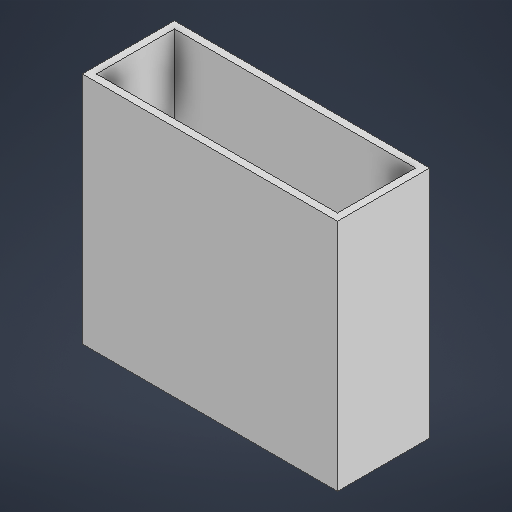
# Autodesk Inventor part: five_cell_bottom_case
Saved by Autodesk Inventor 2026 (Build 300175050, 175E)
## iProperties
Created: 2025-06-13
Part Number: five_cell_bottom_case
Material: Generic
Document SubType Name: Modeling
Designer: hamth
Density: 1 g/cm^3
Appearance: Default
Author: hamth
Autodesk Inventor part; units mm, degrees
ref_plane "YZ Plane" through (0, 0, 0) normal (1, 0, 0) x (0, 1, 0)
ref_plane "XZ Plane" through (0, 0, 0) normal (0, 1, 0) x (-1, 0, 0)
ref_plane "XY Plane" through (0, 0, 0) normal (0, 0, 1) x (1, 0, 0)
sketch "Sketch1" plane through (0, 0, 0) normal (0, 1, 0) x (-1, 0, 0)
  line L0 (57.7037, 0.576) -> (-56.5963, 0.576)
  line L1 (-56.5963, 0.576) -> (-56.5963, 41.851)
  line L2 (-56.5963, 41.851) -> (57.7037, 41.851)
  line L3 (57.7037, 41.851) -> (57.7037, 0.576)
  point P0 (0, 0)
  dimension "d0" = 114.3
  dimension "d1" = 41.275
  constraints: 8 end point, 2 parallel, 1 horizontal, 1 perpendicular
  measures "d0" distance of L1.end L2.end
  measures "d1" distance of L2.end L0.start
extrude "Extrusion1" add sketch "Sketch1" along normal blind 3.175
sketch "Sketch2" plane through (0, 3.175, 0) normal (0, 1, 0) x (1, 0, 0)
  line L0 (56.5963, -0.576) -> (-57.7037, -0.576) projected
  line L1 (-57.7037, -0.576) -> (56.5963, -0.576)
  line L2 (56.5963, -0.576) -> (56.5963, -3.751)
  line L3 (56.5963, -3.751) -> (-57.7037, -3.751)
  line L4 (-57.7037, -3.751) -> (-57.7037, -0.576)
  point P0 (0, 0)
  dimension "d4" = 3.175
  dimension "d5" = 114.3
  constraints: 8 end point, 2 parallel, 1 perpendicular, 1 point on line
  measures "d4" distance of L1.end L2.end
  measures "d5" distance of L2.end L3.end
extrude "Extrusion2" add sketch "Sketch2" along normal blind 101.6
sketch "Sketch3" plane through (0, 3.175, 0) normal (0, 1, 0) x (1, 0, 0)
  line L0 (-57.7037, -41.851) -> (56.5963, -41.851) projected
  line L1 (-57.7037, -41.851) -> (56.5963, -41.851)
  line L2 (56.5963, -41.851) -> (56.5963, -38.676)
  line L3 (56.5963, -38.676) -> (-57.7037, -38.676)
  line L4 (-57.7037, -38.676) -> (-57.7037, -41.851)
  point P0 (0, 0)
  dimension "d8" = 3.175
  dimension "d9" = 114.3
  constraints: 8 end point, 2 parallel, 1 perpendicular, 1 point on line
  measures "d8" distance of L1.end L2.end
  measures "d9" distance of L2.end L3.end
extrude "Extrusion3" add sketch "Sketch3" along normal blind 101.6
sketch "Sketch4" plane through (0, 3.175, 0) normal (0, 1, 0) x (1, 0, 0)
  line L0 (-57.7037, -3.751) -> (-57.7037, -38.676) projected
  line L1 (-57.7037, -3.751) -> (-54.5287, -3.751)
  line L2 (-54.5287, -3.751) -> (-54.5287, -38.676)
  line L3 (-54.5287, -38.676) -> (-57.7037, -38.676)
  line L4 (-57.7037, -38.676) -> (-57.7037, -3.751)
  point P0 (0, 0)
  dimension "d12" = 3.175
  dimension "d13" = 34.925
  constraints: 8 end point, 2 parallel, 2 perpendicular
  measures "d12" distance of L2.end L3.end
  measures "d13" distance of L1.end L2.end
extrude "Extrusion4" add sketch "Sketch4" along normal blind 101.6
sketch "Sketch5" plane through (0, 3.175, 0) normal (0, 1, 0) x (1, 0, 0)
  line L0 (-54.5287, -3.751) -> (56.5963, -3.751) projected
  line L1 (56.5963, -3.751) -> (53.4213, -3.751)
  line L2 (53.4213, -3.751) -> (53.4213, -38.676)
  line L3 (53.4213, -38.676) -> (56.5963, -38.676)
  line L4 (56.5963, -38.676) -> (56.5963, -3.751)
  point P0 (0, 0)
  dimension "d16" = 3.175
  dimension "d17" = 34.925
  constraints: 8 end point, 2 parallel, 1 perpendicular, 1 point on line
  measures "d16" distance of L2.end L3.end
  measures "d17" distance of L1.end L2.end
extrude "Extrusion5" add sketch "Sketch5" along normal blind 101.6
sketch "Sketch6" plane through (0, 3.175, 0) normal (0, 1, 0) x (1, 0, 0)
  line L0 (-54.5287, -38.676) -> (-54.5287, -3.751) projected
  line L1 (-54.5287, -3.751) -> (53.4213, -3.751) projected
  line L2 (-54.5287, -3.751) -> (53.4213, -3.751)
  line L3 (53.4213, -3.751) -> (53.4213, -6.926)
  line L4 (53.4213, -6.926) -> (-54.5287, -6.926)
  line L5 (-54.5287, -6.926) -> (-54.5287, -3.751)
  point P0 (0, 0)
  point P1 (-54.5287, -6.926)
  dimension "d20" = 107.95
  dimension "d21" = 3.175
  constraints: 8 end point, 2 parallel, 1 perpendicular, 1 point on line
  measures "d20" distance of L3.end L4.end
  measures "d21" distance of L2.end L3.end
extrude "Extrusion6" add sketch "Sketch6" along normal blind 12.7
sketch "Sketch7" plane through (0, 3.175, 0) normal (0, 1, 0) x (1, 0, 0)
  line L0 (-54.5287, -38.676) -> (53.4213, -38.676) projected
  line L1 (-54.5287, -38.676) -> (53.4213, -38.676)
  line L2 (53.4213, -38.676) -> (53.4213, -35.501)
  line L3 (53.4213, -35.501) -> (-54.5287, -35.501)
  line L4 (-54.5287, -35.501) -> (-54.5287, -38.676)
  point P0 (0, 0)
  dimension "d24" = 3.175
  dimension "d25" = 107.95
  constraints: 8 end point, 2 parallel, 1 perpendicular, 1 point on line
  measures "d24" distance of L1.end L2.end
  measures "d25" distance of L2.end L3.end
extrude "Extrusion7" add sketch "Sketch7" along normal blind 12.7
sketch "Sketch9" plane through (0, 3.175, 0) normal (0, 1, 0) x (1, 0, 0)
  line L0 (-54.5287, -6.926) -> (53.4213, -6.926) projected
  line L1 (-54.5287, -6.926) -> (-51.3537, -6.926)
  line L2 (-51.3537, -6.926) -> (-51.3537, -35.501)
  line L3 (-51.3537, -35.501) -> (-54.5287, -35.501)
  line L4 (-54.5287, -35.501) -> (-54.5287, -6.926)
  point P0 (0, 0)
  dimension "d30" = 3.175
  dimension "d31" = 28.575
  constraints: 8 end point, 2 parallel, 1 perpendicular, 1 point on line
  measures "d30" distance of L2.end L3.end
  measures "d31" distance of L1.end L2.end
extrude "Extrusion8" add sketch "Sketch9" along normal blind 12.7
sketch "Sketch10" plane through (0, 3.175, 0) normal (0, 1, 0) x (1, 0, 0)
  line L0 (53.4213, -3.751) -> (53.4213, -6.926) projected
  line L1 (-54.5287, -6.926) -> (53.4213, -6.926) projected
  line L2 (53.4213, -6.926) -> (50.2463, -6.926)
  line L3 (50.2463, -6.926) -> (50.2463, -35.501)
  line L4 (50.2463, -35.501) -> (53.4213, -35.501)
  line L5 (53.4213, -35.501) -> (53.4213, -6.926)
  point P0 (0, 0)
  point P1 (-51.3537, -6.926)
  dimension "d34" = 3.175
  dimension "d35" = 28.575
  constraints: 8 end point, 2 parallel, 1 perpendicular, 1 point on line
  measures "d34" distance of L3.end L4.end
  measures "d35" distance of L2.end L3.end
extrude "Extrusion9" add sketch "Sketch10" along normal blind 12.7
sketch "Sketch11" plane through (0, 0, 0) normal (0, -1, 0) x (1, 0, 0)
  line L0 (56.5963, 41.851) -> (56.5963, 0.576) projected
  line L1 (56.5963, 41.851) -> (56.5963, 21.2135)
  line L2 (56.5963, 21.2135) -> (-0.5537, 21.2135)
  point P0 (0, 0)
  dimension "d38" = 20.6375
  dimension "d39" = 57.15
  constraints: 4 end point, 1 midpoint, 1 perpendicular
  measures "d38" distance of L0.start L1.end
  measures "d39" distance of L1.end L2.end
hole "Hole1" at (-0.5537, 0, 21.2135) direction (0, 1, 0) diameter 12.7 end through all
body "Solid1"
